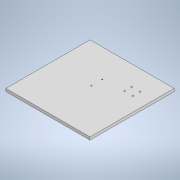
# Autodesk Inventor part: Base
Saved by Autodesk Inventor 2022 (Build 260153000, 153)
## iProperties
Created: 2022-01-01
Part Number: Base
Material: Generic
Document SubType Name: Modeling
Designer: Mlees
Density: 1 g/cm^3
Appearance: Default
Author: Mlees
Autodesk Inventor part; units mm, degrees
ref_plane "YZ Plane" through (0, 0, 0) normal (1, 0, 0) x (0, 1, 0)
ref_plane "XZ Plane" through (0, 0, 0) normal (0, 1, 0) x (-1, 0, 0)
ref_plane "XY Plane" through (0, 0, 0) normal (0, 0, 1) x (1, 0, 0)
sketch "Sketch1" plane through (0, 0, 0) normal (0, 1, 0) x (-1, 0, 0)
  line L0 (0, 0) -> (300, 0)
  line L1 (300, 0) -> (300, -300)
  line L2 (300, -300) -> (0, -300)
  line L3 (0, -300) -> (0, 0)
  dimension "d0" = 300
  dimension "d1" = 300
  constraints: 8 end point, 2 parallel, 1 horizontal, 1 perpendicular
  measures "d0" distance of L1.end L2.end
  measures "d1" distance of L0.end L1.end
extrude "Extrusion1" add sketch "Sketch1" along normal blind 10
sketch "Sketch2" plane through (0, 10, 0) normal (0, 1, 0) x (1, 0, 0)
  line L0 (0, 0) -> (0, 300) projected
  line L1 (0, 150) -> (-50, 150)
  circle A0 centre (-50, 203.3) radius 2.1209
  circle A1 centre (-50, 228.7) radius 2.1209
  circle A2 centre (-79.9974, 203.3) radius 2.1209
  circle A3 centre (-79.9974, 228.7) radius 2.1209
  dimension "d4" = 50
  dimension "d7" = 4.2418
  constraints: 4 centre point, 2 end point, 1 horizontal, 1 midpoint
  measures "d4" distance of L1.start L1.end
  measures "d7" diameter of A0
extrude "Extrusion2" cut sketch "Sketch2" against normal through all
sketch "Sketch3" plane through (0, 10, 0) normal (0, 1, 0) x (1, 0, 0)
  circle A0 centre (-79.9974, 203.3) radius 2.1209 projected
  circle A1 centre (-50, 203.3) radius 2.1209 projected
  line L0 (-79.9974, 203.3) -> (-50, 203.3)
  line L1 (-64.9987, 203.3) -> (-64.9987, 160)
  line L2 (-64.9987, 160) -> (-125.2267, 160)
  line L3 (-125.2267, 160) -> (-155.3807, 160)
  circle A2 centre (-155.3807, 160) radius 2
  circle A3 centre (-155.3805, 199.13) radius 2
  point P0 (0, 0)
  dimension "d12" = 43.3
  dimension "d13" = 60.228
  dimension "d14" = 30.154
  dimension "d15" = 4
  constraints: 8 end point, 2 centre point, 2 horizontal, 1 coincident, 1 midpoint, 1 point on line, 1 vertical
  measures "d12" distance of L1.start L1.end
  measures "d13" distance of L1.end L2.end
  measures "d14" distance of L2.end L3.end
  measures "d15" diameter of A2
extrude "Extrusion3" cut sketch "Sketch3" against normal through all contours A2 | A3
body "Solid1"
